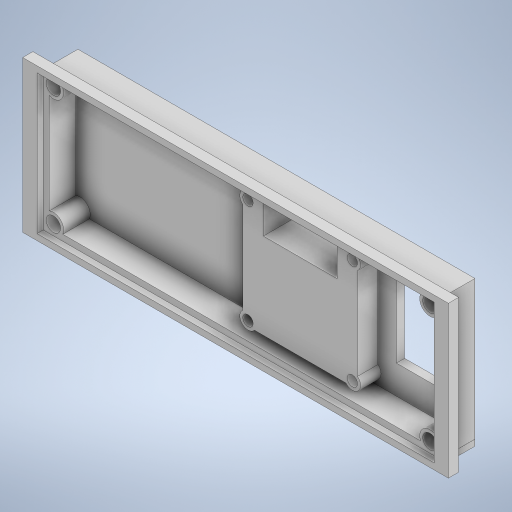
# Autodesk Inventor part: suporte_lcd_botoes
Saved by Autodesk Inventor 2024.3 (Build 283343000, 343)
## iProperties
Created: 2025-02-24
Part Number: suporte_lcd_botoes
Material: Genérico
Document SubType Name: Modeling
Designer: lostv
Density: 1 g/cm^3
Appearance: Padrão
Author: lostv
Autodesk Inventor part; units mm, degrees
ref_plane "YZ Plane" through (0, 0, 0) normal (1, 0, 0) x (0, 1, 0)
ref_plane "XZ Plane" through (0, 0, 0) normal (0, 1, 0) x (-1, 0, 0)
ref_plane "XY Plane" through (0, 0, 0) normal (0, 0, 1) x (1, 0, 0)
sketch "Esboço1" plane through (0, 0, 0) normal (0, 1, 0) x (-1, 0, 0)
  line L0 (-56.5608, 57.9684) -> (47.4498, 57.9684)
  line L1 (47.4498, 57.9684) -> (47.4498, 47.9684)
  line L2 (-56.5608, 47.9684) -> (-56.5608, 57.9684)
  circle A0 centre (-49.5502, 52.951) radius 1.75
  circle A1 centre (40.4498, 52.951) radius 1.75
  circle A2 centre (-4.4961, 52.9684) radius 1.75
  line L3 (37.4498, 47.9684) -> (-46.5502, 47.9684)
  line L4 (43.9498, 47.9684) -> (37.2226, 47.9684)
  line L5 (37.4498, 47.9684) -> (-46.5502, 47.9684)
  line L6 (-53.0502, 47.9684) -> (-46.323, 47.9684)
  line L7 (47.4498, 47.9684) -> (-56.5608, 47.9684)
  line L8 (-53.0502, 47.9684) -> (-53.0502, 57.9684) construction
  line L9 (47.4498, 55.4684) -> (-56.5608, 55.4684)
  line L10 (-53.0502, 47.9684) -> (-53.0502, 57.9684)
  line L11 (43.9498, 47.9684) -> (43.9498, 57.9684)
  point P0 (43.9498, 55.4684)
  point P1 (-53.0502, 55.4684)
  dimension "d4" = 3.5
  dimension "d5" = 5
  dimension "d16" = 2.5
  dimension "d17" = 10
  dimension "d77" = 3.5106
  dimension "d78" = 3.5
  constraints: 24 end point, 6 point on line, 5 horizontal, 3 centre point, 3 perpendicular, 1 collinear, 1 parallel, 1 vertical
  measures "d4" diameter of A2
  measures "d5" distance from line of A2.centre L0
  measures "d16" distance between parallel lines of L9 L0
  measures "d17" distance from line of L1.end L0
  measures "d77" distance between parallel lines of L2 L8
  measures "d78" distance between parallel lines of L11 L1
extrude "Extrusão1" add sketch "Esboço1" along normal blind 37 contours L0 L10 L9 L2 | L0 L11 L9 L10 | L0 L1 L9 L11
extrude "Extrusão2" add sketch "Esboço1" along normal blind 2.5 contours L9 L11 L4 L3 L6 L10
sketch "Esboço2" plane through (-47.4498, 0, 57.9684) normal (0, 0, 1) x (1, 0, 0)
  line L0 (3.5, 35.5) -> (100.5106, 35.5)
  line L1 (100.5106, 35.5) -> (100.5106, 1.5)
  line L2 (100.5106, 1.5) -> (3.5, 1.5)
  line L3 (3.5, 1.5) -> (3.5, 35.5)
  line L4 (0, 0) -> (0, 37) projected
  line L5 (0, 37) -> (104.0106, 37) projected
  line L6 (0, 0) -> (104.0106, 0) projected
  line L7 (104.0106, 0) -> (104.0106, 37) projected
  circle A0 centre (6, 33) radius 1.75
  circle A1 centre (6, 33) radius 2.5
  circle A2 centre (6, 4) radius 1.75
  circle A3 centre (6, 4) radius 2.5
  circle A4 centre (98.0106, 33) radius 2.5
  circle A5 centre (98.0106, 33) radius 1.75
  circle A6 centre (98.0106, 4) radius 2.5
  circle A7 centre (98.0106, 4) radius 1.75
  line L8 (78.8028, 29.8071) -> (78.8028, 7.4296)
  line L9 (21.5, 15.5) -> (31.5, 15.5)
  line L10 (31.5, 15.5) -> (31.5, 5.5)
  line L11 (31.5, 5.5) -> (21.5, 5.5)
  line L12 (21.5, 5.5) -> (21.5, 15.5)
  line L13 (35.5, 23.5) -> (45.5, 23.5)
  line L14 (45.5, 23.5) -> (45.5, 13.5)
  line L15 (45.5, 13.5) -> (35.5, 13.5)
  line L16 (35.5, 13.5) -> (35.5, 23.5)
  line L17 (21.5, 31.5) -> (31.5, 31.5)
  line L18 (31.5, 31.5) -> (31.5, 21.5)
  line L19 (31.5, 21.5) -> (21.5, 21.5)
  line L20 (21.5, 21.5) -> (21.5, 31.5)
  line L21 (7.5, 23.5) -> (17.5, 23.5)
  line L22 (17.5, 23.5) -> (17.5, 13.5)
  line L23 (17.5, 13.5) -> (7.5, 13.5)
  line L24 (7.5, 13.5) -> (7.5, 23.5)
  line L25 (83.324, 30) -> (93.324, 30)
  line L26 (93.324, 30) -> (93.324, 10)
  line L27 (93.324, 10) -> (83.324, 10)
  line L28 (83.324, 10) -> (83.324, 30)
  circle A8 centre (26.5, 26.5) radius 3.5
  circle A9 centre (40.5, 18.5) radius 3.5
  circle A10 centre (26.5, 10.5) radius 3.5
  circle A11 centre (12.5, 18.5) radius 3.5
  line L29 (8.2913, 34) -> (95.7193, 34)
  line L30 (5, 6.2913) -> (5, 30.7087)
  line L31 (95.7193, 3) -> (8.2913, 3)
  line L32 (99.0106, 30.7087) -> (99.0106, 6.2913)
  circle A12 centre (52.0528, 31.3683) radius 1.25
  circle A13 centre (77.5528, 5.8683) radius 1.25
  circle A14 centre (77.5528, 31.3683) radius 1.25
  circle A15 centre (52.0528, 5.8683) radius 1.25
  circle A16 centre (52.0528, 5.8683) radius 2
  circle A17 centre (52.0528, 31.3683) radius 2
  circle A18 centre (77.5528, 31.3683) radius 2
  circle A19 centre (77.5528, 5.8683) radius 2
  line L33 (55.8028, 32.6183) -> (73.8028, 32.6183)
  line L34 (73.8028, 32.6183) -> (73.8028, 25.6183)
  line L35 (73.8028, 25.6183) -> (55.8028, 25.6183)
  line L36 (55.8028, 25.6183) -> (55.8028, 32.6183)
  line L37 (50.8028, 7.4296) -> (50.8028, 29.8071)
  line L38 (50.8028, 31.3683) -> (50.8028, 31.5)
  line L39 (53.6141, 32.6183) -> (75.9916, 32.6183)
  line L40 (78.8028, 4.6183) -> (77.5528, 4.6183)
  line L41 (75.9916, 4.6183) -> (53.6141, 4.6183)
  line L42 (52.0528, 4.6183) -> (50.8028, 4.6183)
  point P0 (47.4498, 0)
  point P1 (26.5, 15.5)
  point P2 (64.8028, 25.6183)
  point P3 (64.8028, 32.6183)
  dimension "d81" = 2.5
  dimension "d82" = 2.5
  dimension "d84" = 2.5
  dimension "d22" = 3.5
  dimension "d23" = 1.5
  dimension "d24" = 1.5
  dimension "d25" = 3.5
  dimension "d26" = 3.5
  dimension "d27" = 5
  dimension "d28" = 3.5
  dimension "d29" = 5
  dimension "d30" = 5
  dimension "d31" = 3.5
  dimension "d32" = 5
  dimension "d33" = 3.5
  dimension "d34" = 104.0106
  dimension "d35" = 37
  dimension "d36" = 28
  dimension "d38" = 10
  dimension "d39" = 10
  dimension "d40" = 10
  dimension "d41" = 10
  dimension "d42" = 10
  dimension "d43" = 10
  dimension "d44" = 10
  dimension "d45" = 10
  dimension "d46" = 10
  dimension "d47" = 20
  dimension "d48" = 4
  dimension "d49" = 4
  dimension "d50" = 4
  dimension "d51" = 4
  dimension "d52" = 4
  dimension "d53" = 4
  dimension "d54" = 4
  dimension "d55" = 12
  dimension "d56" = 12
  dimension "d57" = 5.5
  dimension "d58" = 7
  dimension "d59" = 7
  dimension "d60" = 7
  dimension "d61" = 7
  dimension "d65" = 1.5
  dimension "d72" = 6
  dimension "d83" = 2.5
  dimension "d85" = 4
  dimension "d86" = 4
  dimension "d87" = 4
  dimension "d88" = 4
  dimension "d90" = 5
  dimension "d91" = 7
  constraints: 78 end point, 21 parallel, 17 centre point, 16 point on circle, 13 horizontal, 9 perpendicular, 8 coincident, 8 tangent, 3 midpoint, 3 vertical, 2 point on line, 2 vertical alignment, 1 horizontal alignment, 6 other
  measures "d22" distance between parallel lines of L4 L3
  measures "d23" distance between parallel lines of L5 L0
  measures "d24" distance between parallel lines of L6 L2
  measures "d25" distance between parallel lines of L7 L1
  measures "d26" diameter of A0
  measures "d27" diameter of A1
  measures "d28" diameter of A2
  measures "d29" diameter of A3
  measures "d30" diameter of A4
  measures "d31" diameter of A5
  measures "d32" diameter of A6
  measures "d33" diameter of A7
  measures "d34" distance between parallel lines of L7 L4
  measures "d35" distance between parallel lines of L6 L5
  measures "d36" distance of L40.start L42.end
  measures "d38" distance of L10.end L11.end
  measures "d39" distance of L9.end L10.end
  measures "d40" distance of L14.end L16.start
  measures "d41" distance of L14.start L14.end
  measures "d42" distance of L18.end L20.start
  measures "d43" distance of L18.start L18.end
  measures "d44" distance of L22.end L24.start
  measures "d45" distance of L22.start L22.end
  measures "d46" distance of L26.end L27.end
  measures "d47" distance between parallel lines of L27 L25
  measures "d48" distance between parallel lines of L3 L24
  measures "d49" distance between parallel lines of L22 L20
  measures "d50" distance between parallel lines of L22 L12
  measures "d51" distance between parallel lines of L10 L16
  measures "d52" distance between parallel lines of L18 L16
  measures "d53" distance between parallel lines of L2 L11
  measures "d54" distance between parallel lines of L0 L17
  measures "d55" distance between parallel lines of L2 L23
  measures "d56" distance between parallel lines of L13 L0
  measures "d57" distance between parallel lines of L0 L25
  measures "d58" diameter of A8
  measures "d59" diameter of A9
  measures "d60" diameter of A10
  measures "d61" diameter of A11
  measures "d65" distance between parallel lines of L0 L29
  measures "d72" distance from line of point (26.5, 15.5) L19
  measures "d83" diameter of A14
  measures "d85" diameter of A16
  measures "d86" diameter of A17
  measures "d87" diameter of A18
  measures "d88" diameter of A19
  measures "d90" distance between parallel lines of L8 L34
  measures "d91" distance of point (64.803, 25.618) point (64.803, 32.618)
extrude "Extrusão3" add sketch "Esboço2" against normal blind 10 contours L0 A1 L3 | L0 A4 L29 A1 | A1 | A1 L30 A3 L3 | L0 L1 A4 | A4 | L29 A4 L32 A6 L31 A3 L30 A1 | A3 L2 L3 | A3 | L1 A6 L32 A4 | A3 L31 A6 L2 | A6 | L1 L2 A6 | A0 | A2 | A5 | A7 | L8 A19 L41 A16 L37 A17 L39 L36 L35 L34 A18 | A18 | A19 | L34 L35 L36 L33 | A16 | A17 | L9 L10 L11 L12 | L13 L14 L15 L16 | L17 L18 L19 L20 | L21 L22 L23 L24 | L25 L26 L27 L28 | A8 | A9 | A10 | A11 | A12 | A13 | A14 | A15
extrude "Extrusão4" cut sketch "Esboço2" against normal blind 8 contours L29 A4 L32 A6 L31 A3 L30 A1 | L8 A19 L41 A16 L37 A17 L39 L36 L35 L34 A18 | A18 | A19 | L34 L35 L36 L33 | A16 | A17 | L9 L10 L11 L12 | L13 L14 L15 L16 | L17 L18 L19 L20 | L21 L22 L23 L24 | L25 L26 L27 L28 | A8 | A9 | A10 | A11 | A12 | A13 | A14 | A15
extrude "Extrusão5" cut sketch "Esboço2" against normal blind 1.5 contours L0 A1 L3 | L0 A4 L29 A1 | A1 | A1 L30 A3 L3 | L0 L1 A4 | A4 | A3 L2 L3 | A3 | L1 A6 L32 A4 | A3 L31 A6 L2 | A6 | L1 L2 A6 | A0 | A2 | A5 | A7
extrude "Extrusão6" cut sketch "Esboço2" against normal blind 8 contours A0 | A2 | A5 | A7
extrude "Extrusão7" cut sketch "Esboço2" against normal through all contours L25 L26 L27 L28
extrude "Extrusão8" cut sketch "Esboço1" along normal blind 2 contours A0 | A1 | A2
extrude "Extrusão9" add sketch "Esboço2" against normal blind 8.5 contours L8 A19 L41 A16 L37 A17 L39 L36 L35 L34 A18 | A18 | A19 | A16 | A17
extrude "Extrusão10" cut sketch "Esboço2" against normal blind 3 contours L8 A19 L41 A16 L37 A17 L39 L36 L35 L34 A18 | A18 | A19 | A16 | A17 | A13 | A14 | A15
extrude "Extrusão11" cut sketch "Esboço2" against normal through all contours L34 L35 L36 L33
